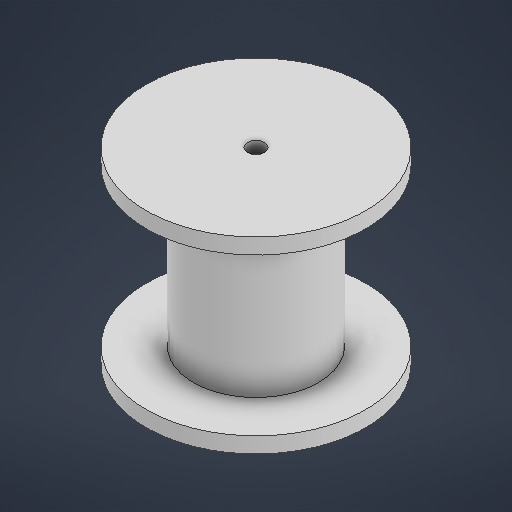
# Autodesk Inventor part: spool2
Saved by Autodesk Inventor 2027 (Build 310192060, 192F)
## iProperties
Created: 2026-06-15
Part Number: spool2
Material: Generic
Document SubType Name: Modeling
Designer: beave
Density: 1 g/cm^3
Appearance: Default
Author: beave
Autodesk Inventor part; units mm, degrees
ref_plane "YZ Plane" through (0, 0, 0) normal (1, 0, 0) x (0, 1, 0)
ref_plane "XZ Plane" through (0, 0, 0) normal (0, 1, 0) x (-1, 0, 0)
ref_plane "XY Plane" through (0, 0, 0) normal (0, 0, 1) x (1, 0, 0)
sketch "Sketch9" plane through (0, 0, 0) normal (0, 1, 0) x (-1, 0, 0)
  circle A0 centre (0, 0) radius 20
  circle A1 centre (0, 0) radius 35
  dimension "d43" = 40
  dimension "d44" = 70
  constraints: 2 centre point, 1 coincident
  measures "d43" diameter of A0
  measures "d44" diameter of A1
extrude "Extrusion4" add sketch "Sketch9" along normal blind 5
sketch "Sketch10" plane through (0, 0, 0) normal (0, -1, 0) x (1, 0, 0)
  circle A0 centre (0, 0) radius 20
  dimension "d47" = 40
  constraints: 1 centre point, 1 coincident
  measures "d47" diameter of A0
extrude "Extrusion5" add sketch "Sketch10" against normal blind 60
mirror "Mirror2" about plane through (0, 0, 0) normal (0, 1, 0) bodies 1 separate body
move or copy body "Move Body7" bodies to move or copy 2 copy no translate (0, 60, 0)
combine bodies "Combine2" operation type add bodies to combine 1 2
sketch "Sketch11" plane through (0, 60, 0) normal (0, 1, 0) x (1, 0, 0)
  circle A0 centre (0, 0) radius 35 projected
  constraints: 1 coincident
hole "Hole3" at (0, 60, 0) direction (0, -1, 0) diameter 32 end through all bodies 1
sketch "Sketch13" plane through (0, 55, 0) normal (0, -1, 0) x (1, 0, 0)
  circle A0 centre (0, 0) radius 19.5
  dimension "d64" = 39
  constraints: 1 centre point, 1 coincident
  measures "d64" diameter of A0
extrude "Extrusion6" add sketch "Sketch13" against normal blind 5 bodies 1
sketch "Sketch15" plane through (0, 55, 0) normal (0, -1, 0) x (1, 0, 0)
  circle A0 centre (0, 0) radius 19
  dimension "d74" = 38
  constraints: 1 centre point, 1 coincident
  measures "d74" diameter of A0
extrude "Extrusion7" add sketch "Sketch15" along normal blind 2 bodies 1
sketch "Sketch18" plane through (0, 53, 0) normal (0, -1, 0) x (1, 0, 0)
  circle A0 centre (-1.2742, 0.7124) radius 19.5
  point P0 (0, 0)
  dimension "d85" = 39
  constraints: 1 centre point
  measures "d85" diameter of A0
extrude "Extrusion8" add sketch "Sketch18" along normal blind 0.5 bodies 1
sketch "Sketch19" plane through (0, 60, 0) normal (0, 1, 0) x (1, 0, 0)
  circle A0 centre (0, 0) radius 35 projected
  constraints: 1 coincident
hole "Hole6" at (0, 60, 0) direction (0, -1, 0) diameter 5.5 end through all bodies 1 clearance for "Flat Head Machine Screw" size "M5" standard "Ansi Metric M Profile"
body "Solid3"
